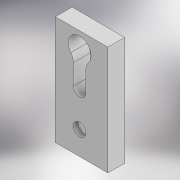
# Autodesk Inventor part: Prueba3D
Saved by Autodesk Inventor 2021 (Build 250183000, 183)
## iProperties
Created: 2024-02-25
Part Number: Prueba3D
Material: Generic
Document SubType Name: Modeling
Designer: Martin
Density: 1 g/cm^3
Appearance: Default
Author: Martin
Autodesk Inventor part; units mm, degrees
ref_plane "YZ Plane" through (0, 0, 0) normal (1, 0, 0) x (0, 1, 0)
ref_plane "XZ Plane" through (0, 0, 0) normal (0, 1, 0) x (-1, 0, 0)
ref_plane "XY Plane" through (0, 0, 0) normal (0, 0, 1) x (1, 0, 0)
sketch "Sketch1" plane through (0, 0, 0) normal (0, 0, 1) x (1, 0, 0)
  circle A0 centre (0, 9.4768) radius 4.1
  circle A1 centre (0, 9.4768) radius 11.1
  arc A2 (5.7519, 50.2372) -> (4.0065, 45.5517) centre (13.9526, 44.5146) ccw
  arc A3 (-3.9935, 45.5517) -> (-5.7388, 50.2372) centre (-13.9395, 44.5146) ccw
  line L0 (4.0065, 55.0581) -> (4.0065, 33.0581)
  line L1 (-3.9935, 33.0581) -> (-3.9935, 55.0581)
  line L2 (-3.9935, 55.0581) -> (4.0065, 55.0581)
  line L3 (0.0065, 55.0581) -> (5.7519, 50.2372)
  line L4 (0.0065, 55.0581) -> (0.0065, 47.5581) construction
  line L5 (0.0065, 55.0581) -> (-5.7388, 50.2372)
  circle A4 centre (0.0065, 55.0581) radius 7.5
  line L6 (4.0065, 33.0581) -> (-3.9935, 33.0581)
  line L7 (0.0065, 55.0581) -> (0.0065, 32.0581) construction
  line L8 (4.0065, 55.0581) -> (4.0065, 32.0581)
  line L9 (-3.9935, 32.0581) -> (-3.9935, 55.0581)
  arc A5 (4.0065, 55.0581) -> (-3.9935, 55.0581) centre (0.0065, 55.0581) ccw
  arc A6 (-3.9935, 32.0581) -> (4.0065, 32.0581) centre (0.0065, 32.0581) ccw
  line L10 (-15.9677, -6.0429) -> (18.5773, -6.0429)
  line L11 (18.5773, -6.0429) -> (18.5773, 65.522)
  line L12 (18.5773, 65.522) -> (-15.9677, 65.522)
  line L13 (-15.9677, 65.522) -> (-15.9677, -6.0429)
  point P0 (0, 0)
  point P1 (0.0065, 55.0581)
  point P2 (0.0065, 55.0581)
  point P3 (0.0065, 43.5581)
  point P4 (-3.9935, 45.5517)
  dimension "d2" = 15
  dimension "d0" = 8.2
  dimension "d1" = 22.2
  dimension "d3" = 22
  dimension "d4" = 8
  dimension "d5" = 50
  dimension "d6" = 5
  dimension "d7" = 10
  dimension "d8" = 23
  constraints: 30 end point, 8 point on circle, 6 centre point, 5 parallel, 4 tangent, 2 perpendicular, 1 coincident, 1 equal length, 1 horizontal, 1 midpoint, 1 point on line, 3 other
  measures "d0" diameter of A0
  measures "d1" diameter of A1
  measures "d3" distance of L6.end L2.start
  measures "d4" distance of L6.start L6.end
  measures "d5" angle of L4 L3
  measures "d6" distance of L3.end A2.end
  measures "d7" radius of A2
  measures "d8" distance of L7.start L7.end
extrude "Extrusion1" add sketch "Sketch1" along normal blind 3 contours A1 | L13 L12 L11 L10
extrude "Extrusion2" add sketch "Sketch1" against normal blind 8 contours L13 L12 L11 L10
body "Solid1"
